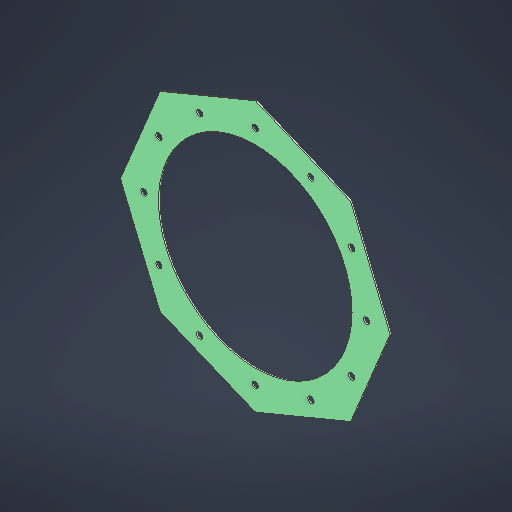
# Autodesk Inventor part: DMF 01 21 Барабан торец НОС v2.1
Saved by Autodesk Inventor 2026.2 (Build 302298010, 298A)
## iProperties
Created: 2024-04-28
Part Number: DMF 01 21 Барабан торец НОС v2.1
Material: Generic
Document SubType Name: Sheet Metal
Designer: pokla
Density: 1 g/cm^3
Appearance: Default
Sheet Metal Rule: Default
Flat Pattern Width: 51.5 cm
Flat Pattern Length: 51.5 cm
Flat Pattern Area: 2652.25 cm^2
Sheet Metal Width: 515,000 mm
Sheet Metal Length: 515,000 mm
Sheet Metal Area: 265225,000 mm^2
Stock Number: Барабан_Торец_Нос
Author: pokla
Autodesk Inventor part; units mm, degrees
ref_plane "YZ Plane" through (0, 0, 0) normal (1, 0, 0) x (0, 1, 0)
ref_plane "XZ Plane" through (0, 0, 0) normal (0, 1, 0) x (-1, 0, 0)
ref_plane "XY Plane" through (0, 0, 0) normal (0, 0, 1) x (1, 0, 0)
sketch "Sketch2" plane through (0, 0, 0) normal (0, 0, 1) x (1, 0, 0)
  line L0 (-197.082, 197.082) -> (0, 278.716)
  line L1 (0, 278.716) -> (197.082, 197.082)
  line L2 (197.082, 197.082) -> (278.716, 0)
  line L3 (278.716, 0) -> (197.082, -197.082)
  line L4 (197.082, -197.082) -> (0, -278.716)
  line L5 (0, -278.716) -> (-197.082, -197.082)
  line L6 (-197.082, -197.082) -> (-278.716, 0)
  line L7 (-278.716, 0) -> (-197.082, 197.082)
  circle A0 centre (0, 0) radius 200
  dimension "d23" = 515
  dimension "d26" = 400
  measures "d23" distance between parallel lines of L6 L2
  measures "d26" diameter of A0
extrude "Plate1" add sketch "Sketch2" against normal blind 3
sketch "Sketch4" plane through (0, 0, 0) normal (0, 0, 1) x (1, 0, 0)
  circle A0 centre (0, 230) radius 6.5
  circle A1 centre (0, 0) radius 200 construction
  circle A2 centre (0, 0) radius 230 construction
  circle A3 centre (-115, 199.1858) radius 6.5
  circle A4 centre (-199.1858, 115) radius 6.5
  circle A5 centre (-230, 0) radius 6.5
  circle A6 centre (-199.1858, -115) radius 6.5
  circle A7 centre (-115, -199.1858) radius 6.5
  circle A8 centre (0, -230) radius 6.5
  circle A9 centre (115, -199.1858) radius 6.5
  circle A10 centre (199.1858, -115) radius 6.5
  circle A11 centre (230, 0) radius 6.5
  circle A12 centre (199.1858, 115) radius 6.5
  circle A13 centre (115, 199.1858) radius 6.5
  dimension "d32" = 460
  dimension "d16" = 13
  dimension "d30" = 360
  constraints: 12 centre point, 2 vertical alignment, 1 coincident, 27 other
  measures "d16" diameter of A0
extrude "Extrusion1" cut sketch "Sketch4" against normal up to surface (3 mm away)
equation "\"d23\" = Барабан_размер_по_плоскостям"
equation "\"d15\" = Thickness"
equation "\"BendRadius\" = Thickness"
equation "\"BendReliefWidth\" = Thickness"
equation "\"BendReliefDepth\" = 0.5 * Thickness"
equation "\"CornerReliefSize\" = 4 * Thickness"
equation "\"MinimumRemnant\" = 2 * Thickness"
equation "\"TransitionRadius\" = BendRadius"
equation "\"JacobiRadiusSize\" = BendRadius"
equation "\"GapSize\" = Thickness"
equation "\"Барабан_размер_по_плоскостям\" = 515"
equation "\"Thickness\" = 3"
body "Solid1"
